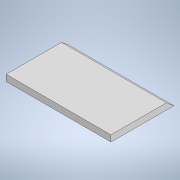
# Autodesk Inventor part: nozz
Saved by Autodesk Inventor 2022 (Build 260153000, 153)
## iProperties
Created: 2023-01-27
Part Number: nozz
Material: Generic
Document SubType Name: Modeling
Designer: Kamil
Density: 1 g/cm^3
Appearance: Default
Author: Kamil
Autodesk Inventor part; units mm, degrees
ref_plane "YZ Plane" through (0, 0, 0) normal (1, 0, 0) x (0, 1, 0)
ref_plane "XZ Plane" through (0, 0, 0) normal (0, 1, 0) x (-1, 0, 0)
ref_plane "XY Plane" through (0, 0, 0) normal (0, 0, 1) x (1, 0, 0)
sketch "Sketch1" plane through (0, 0, 0) normal (1, 0, 0) x (0, 1, 0)
  line L0 (1.944, 4.8709) -> (-1.056, 4.8709)
  line L1 (-1.056, 4.8709) -> (-1.056, -25.1291)
  line L2 (-1.056, -25.1291) -> (1.944, -25.1291)
  line L3 (1.944, -25.1291) -> (1.944, 4.8709)
  line L4 (-1.056, -25.1291) -> (9.6963, -12.315)
  point P0 (0, 0)
  point P1 (1.944, -21.5539)
  dimension "d0" = 3
  dimension "d1" = 30
  dimension "d2" = 40
  constraints: 10 end point, 2 parallel, 1 horizontal, 1 perpendicular
  measures "d0" distance of L2.end L1.end
  measures "d1" distance of L1.end L0.end
  measures "d2" angle of L1 L4
extrude "Extrusion1" add sketch "Sketch1" against normal blind 50 contours L3 L4 L1 L0
body "Solid1"
